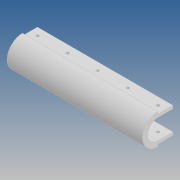
# Autodesk Inventor part: 000.002 - bamper
Saved by Autodesk Inventor 2020 (Build 240168000, 168)
## iProperties
Created: 2021-06-26
Part Number: 000.002 - bamper
Material: Типовые
Document SubType Name: Modeling
Designer: Петров Иван
Mass: 94.863 g
Surface Area: 372.497 cm^2
Volume: 94.863 cm^3
Density: 1 g/cm^3
Appearance: По умолчанию
Author: Петров Иван
Autodesk Inventor part; units mm, degrees
ref_plane "YZ Plane" through (0, 0, 0) normal (1, 0, 0) x (0, 1, 0)
ref_plane "XZ Plane" through (0, 0, 0) normal (0, 1, 0) x (-1, 0, 0)
ref_plane "XY Plane" through (0, 0, 0) normal (0, 0, 1) x (1, 0, 0)
sketch "Эскиз1" plane through (0, 0, 0) normal (0, 1, 0) x (-1, 0, 0)
  line L0 (-90, 10) -> (90, 10)
  line L1 (90, 10) -> (90, -10)
  line L2 (90, -10) -> (-90, -10)
  line L3 (-90, -10) -> (-90, 10)
  line L4 (-90, 10) -> (90, -10) construction
  line L5 (90, 10) -> (-90, -10) construction
  point P0 (0, 0)
  dimension "d0" = 180
  dimension "d1" = 20
  constraints: 12 end point, 2 midpoint, 2 parallel, 1 horizontal, 1 perpendicular
  measures "d0" distance of L1.end L2.end
  measures "d1" distance of L0.end L1.end
extrude "Выдавливание1" add sketch "Эскиз1" along normal blind 4
sketch "Эскиз2" plane through (90, 0, 10) normal (1, 0, 0) x (0, 0, -1)
  line L0 (0, 0) -> (20, 0) projected
  line L1 (0, 0) -> (0, 4) projected
  line L2 (0, 4) -> (20, 4) projected
  arc A0 (-13.3163, 17.3163) -> (0, 4) centre (0, 17.3163) ccw
  arc A1 (-20.3163, 17.3163) -> (0, -3) centre (0, 17.3163) ccw
  line L3 (0, 0) -> (0, -3)
  line L4 (-13.3163, 17.3163) -> (-20.3163, 17.3163)
  point P0 (10, 0)
  point P1 (0, 2)
  dimension "d4" = 3
  constraints: 5 end point, 4 point on circle, 2 centre point, 1 coincident, 1 midpoint, 1 vertical, 1 other
  measures "d4" distance from line of L0 L3.end
extrude "Выдавливание2" add sketch "Эскиз2" against normal blind 180
sketch "Эскиз3" plane through (0, 4, 0) normal (0, 1, 0) x (1, 0, 0)
  circle A0 centre (-80, 0) radius 2
  line L0 (-90, 10) -> (-90, -10) projected
  line L1 (90, 10) -> (-90, 10) projected
  point P0 (0, 0)
  dimension "d7" = 4
  dimension "d8" = 10
  dimension "d9" = 10
  constraints: 1 centre point
  measures "d7" diameter of A0
  measures "d8" distance from line of L0 A0.centre
  measures "d9" distance from line of L1 A0.centre
extrude "Выдавливание3" cut sketch "Эскиз3" against normal blind 180
pattern_linear "Прямоуг.массив1" count 5 spacing 40 along (1, 0, 0) of "Выдавливание3"
mirror "Зеркальное отражение1" about plane through (90, 17.3163, 30.3163) normal (0, 1, 0) of "Выдавливание1", "Выдавливание2", "Выдавливание3", "Прямоуг.массив1"
